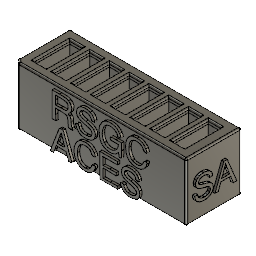
Bargraph Updated 8 Pin (Autodesk Fusion 360 design; units mm, degrees)
Autodesk Fusion 360 part; units mm, degrees
note: some values were not read from the file. Chosen so that the rebuilt part matches the saved one: which face or edge a step refers to; which pieces of a blend or face edit are solid. Set by a fixed rule: which sketch regions a step uses.
(part 1 of 2)
sketch "Sketch2" plane through (0, 0, 0) normal (0, 0, 1) x (-1, 0, 0)
  line L0 (0, -5.1) -> (-2.1, -5.1)
  line L1 (-2.1, -5.1) -> (-2.1, 0)
  line L2 (-2.1, 0) -> (0, 0)
  line L3 (0, 0) -> (0, -5.1)
  line L4 (-2.54, -5.1) -> (-2.54, 0)
  line L5 (-4.64, -5.1) -> (-2.54, -5.1)
  line L6 (-4.64, 0) -> (-4.64, -5.1)
  line L7 (-2.54, 0) -> (-4.64, 0)
  line L8 (-1.05, -2.55) -> (-1.05, -1.28)
  line L9 (-1.05, -2.55) -> (-1.05, -3.82)
  line L10 (-1.05, -3.82) -> (-3.59, -3.82)
  line L11 (-7.62, 0) -> (-9.72, 0)
  line L12 (-5.08, -5.1) -> (-7.18, -5.1)
  line L13 (-7.18, 0) -> (-5.08, 0)
  line L14 (-7.18, -5.1) -> (-7.18, 0)
  line L15 (-7.62, -5.1) -> (-7.62, 0)
  line L16 (-9.72, 0) -> (-9.72, -5.1)
  line L17 (-9.72, -5.1) -> (-7.62, -5.1)
  line L18 (-5.08, 0) -> (-5.08, -5.1)
  line L19 (-7.18, -2.55) -> (-6.13, -2.55)
  line L20 (-6.13, -2.55) -> (-6.13, -3.82)
  line L21 (-3.59, -3.82) -> (-6.13, -3.82)
  line L22 (-9.72, -2.55) -> (-8.67, -2.55)
  line L23 (-8.67, -2.55) -> (-8.67, -3.82)
  line L24 (-8.67, -3.82) -> (-11.21, -3.82)
  line L25 (-12.26, -5.1) -> (-12.26, 0)
  line L26 (-16.29, -2.55) -> (-16.29, -3.82)
  line L27 (-11.21, -3.82) -> (-13.75, -3.82)
  line L28 (-17.78, 0) -> (-19.88, 0)
  line L29 (-17.34, -2.55) -> (-16.29, -2.55)
  line L30 (-19.88, 0) -> (-19.88, -5.1)
  line L31 (-14.8, 0) -> (-14.8, -5.1)
  line L32 (-17.34, -5.1) -> (-17.34, 0)
  line L33 (-12.7, 0) -> (-14.8, 0)
  line L34 (-11.21, -2.55) -> (-11.21, -3.82)
  line L35 (-10.16, -5.1) -> (-12.26, -5.1)
  line L36 (-15.24, -5.1) -> (-17.34, -5.1)
  line L37 (-15.24, 0) -> (-15.24, -5.1)
  line L38 (-14.8, -5.1) -> (-12.7, -5.1)
  line L39 (-12.7, -5.1) -> (-12.7, 0)
  line L40 (-17.34, 0) -> (-15.24, 0)
  line L41 (-10.16, 0) -> (-10.16, -5.1)
  line L42 (-11.21, -2.55) -> (-11.21, -1.28)
  line L43 (-13.75, -3.82) -> (-16.29, -3.82)
  line L44 (-17.78, -5.1) -> (-17.78, 0)
  line L45 (-12.26, 0) -> (-10.16, 0)
  line L46 (-19.88, -5.1) -> (-17.78, -5.1)
  line L47 (-18.83, -2.55) -> (-18.83, -3.82)
  line L48 (-19.88, -2.55) -> (-18.83, -2.55)
  line L49 (0, 0) -> (0, 1)
  line L50 (0, 1) -> (1, 1)
  line L51 (-20.04, -5.1) -> (-21.04, -5.1)
  line L52 (-21.04, -5.1) -> (-21.04, -6.1)
  line L53 (-21.04, -6.1) -> (1, -6.1)
  line L54 (1, -6.1) -> (1, 1)
  line L55 (1, 1) -> (-21.04, 1)
  line L56 (-21.04, 1) -> (-21.04, -6.1)
  line L57 (0.5, 0.5) -> (-20.54, 0.5)
  line L58 (-20.54, 0.5) -> (-20.54, -5.6)
  line L59 (-20.54, -5.6) -> (0.5, -5.6)
  line L60 (0.5, -5.6) -> (0.5, 0.5)
  point P0 (-21.37, -3.82)
  point P1 (-26.45, -3.82)
  point P2 (-26.45, -3.82)
  dimension "d8" = 2.1
  dimension "d9" = 5.1
  dimension "d18" = 1.27
  dimension "d19" = 1.27
  dimension "d29" = 1.05
  dimension "d30" = 2.54
  dimension "d31" = 1.05
  dimension "d32" = 2.54
  dimension "d33" = 2.1
  dimension "d34" = 5.1
  dimension "d35" = 1.27
  dimension "d36" = 1.27
  dimension "d37" = 1.05
  dimension "d38" = 2.54
  dimension "d39" = 1.05
  dimension "d46" = 1
  dimension "d47" = 1
  dimension "d48" = 1
  dimension "d49" = 1
  dimension "d92" = -0.5
  dimension "d95" = 21.04
  dimension "d96" = 6.1
  constraint horizontal L0
  constraint vertical L1
  constraint horizontal L2
  constraint vertical L3
  constraint perpendicular L2 L8
  constraint parallel L8 L9
  constraint perpendicular L4 L10
  constraint horizontal L12
  constraint vertical L14
  constraint horizontal L13
  constraint vertical L18
  constraint midpoint L14 L19.start
  constraint perpendicular L18 L19
  constraint perpendicular L10 L20
  constraint perpendicular L18 L21
  constraint midpoint L16 L22.start
  constraint perpendicular L16 L22
  constraint perpendicular L21 L23
  constraint perpendicular L23 L24
  constraint horizontal L35
  constraint vertical L25
  constraint horizontal L45
  constraint vertical L41
  constraint perpendicular L42 L45
  constraint parallel L34 L42
  constraint perpendicular L27 L39
  constraint horizontal L36
  constraint vertical L32
  constraint horizontal L40
  constraint vertical L37
  constraint midpoint L29.start L32
  constraint perpendicular L29 L37
  constraint perpendicular L26 L27
  constraint perpendicular L37 L43
  constraint midpoint L48.start L30
  constraint perpendicular L30 L48
  constraint perpendicular L43 L47
  constraint perpendicular L2 L49
  constraint perpendicular L3 L50
  constraint horizontal L53
  constraint vertical L54
  constraint horizontal L55
  constraint vertical L56
  measures "d8" distance of L0.start L0.end
  measures "d9" distance of L0.start L2.end
  measures "d18" distance of L8.start L8.end
  measures "d19" distance of L8.start L9.end
  measures "d29" distance of L19.start L19.end
  measures "d30" distance of L10.end L20.end
  measures "d31" distance of L22.start L22.end
  measures "d32" distance of L23.end L24.end
  measures "d33" distance of L35.start L25.start
  measures "d34" distance of L35.start L41.start
  measures "d35" distance of L42.end L34.start
  measures "d36" distance of L24.end L34.start
  measures "d37" distance of L26.start L29.start
  measures "d38" distance of L27.end L26.end
  measures "d39" distance of L48.start L47.start
  measures "d46" distance of L2.end L49.end
  measures "d47" distance of L49.end L50.end
  measures "d48" distance of L51.start L51.end
  measures "d49" distance of L51.end L52.end
  measures "d95" distance of L57.start L57.end
  measures "d96" distance of L57.start L59.end
extrude "Extrude5" add sketch "Sketch2" along normal blind 7.5
sketch "Sketch5" plane through (0, 0, 7.5) normal (0, 0, 1) x (-1, 0, 0)
  line L0 (-17.78, -5.1) -> (-19.88, -5.1)
  line L1 (-19.88, -5.1) -> (-19.88, 0)
  line L2 (-19.88, 0) -> (-17.78, 0)
  line L3 (-17.78, 0) -> (-17.78, -5.1)
  line L4 (-7.18, 0) -> (-5.08, 0)
  line L5 (-5.08, 0) -> (-5.08, -5.1)
  line L6 (-5.08, -5.1) -> (-7.18, -5.1)
  line L7 (-7.18, -5.1) -> (-7.18, 0)
  line L8 (-2.1, 0) -> (0, 0)
  line L9 (0, 0) -> (0, -5.1)
  line L10 (0, -5.1) -> (-2.1, -5.1)
  line L11 (-2.1, -5.1) -> (-2.1, 0)
  line L12 (-17.34, -5.1) -> (-17.34, 0)
  line L13 (-17.34, 0) -> (-15.24, 0)
  line L14 (-15.24, 0) -> (-15.24, -5.1)
  line L15 (-15.24, -5.1) -> (-17.34, -5.1)
  line L16 (-12.7, 0) -> (-12.7, -5.1)
  line L17 (-12.7, -5.1) -> (-14.8, -5.1)
  line L18 (-14.8, -5.1) -> (-14.8, 0)
  line L19 (-14.8, 0) -> (-12.7, 0)
  line L20 (-12.26, -5.1) -> (-12.26, 0)
  line L21 (-12.26, 0) -> (-10.16, 0)
  line L22 (-10.16, 0) -> (-10.16, -5.1)
  line L23 (-10.16, -5.1) -> (-12.26, -5.1)
  line L24 (-7.62, -5.1) -> (-9.72, -5.1)
  line L25 (-9.72, -5.1) -> (-9.72, 0)
  line L26 (-9.72, 0) -> (-7.62, 0)
  line L27 (-7.62, 0) -> (-7.62, -5.1)
  line L28 (-4.64, 0) -> (-2.54, 0)
  line L29 (-2.54, 0) -> (-2.54, -5.1)
  line L30 (-2.54, -5.1) -> (-4.64, -5.1)
  line L31 (-4.64, -5.1) -> (-4.64, 0)
  line L32 (-21.04, 1) -> (-21.04, -6.1)
  line L33 (-21.04, -6.1) -> (1, -6.1)
  line L34 (1, -6.1) -> (1, 1)
  line L35 (1, 1) -> (-21.04, 1)
  line L36 (-18.83, -2.55) -> (-16.29, -2.55)
  line L37 (-16.29, -2.55) -> (-13.75, -2.55)
  line L38 (-13.75, -2.55) -> (-11.21, -2.55)
  line L39 (-11.21, -2.55) -> (-8.67, -2.55)
  line L40 (-8.67, -2.55) -> (-6.13, -2.55)
  line L41 (-6.13, -2.55) -> (-3.59, -2.55)
  line L42 (-3.59, -2.55) -> (-1.05, -2.55)
  line L43 (-0.25, -4.85) -> (-1.85, -4.85)
  line L44 (-1.85, -4.85) -> (-1.85, -0.25)
  line L45 (-1.85, -0.25) -> (-0.25, -0.25)
  line L46 (-0.25, -0.25) -> (-0.25, -4.85)
  line L47 (-0.25, -4.85) -> (-1.85, -0.25) construction
  line L48 (-1.85, -4.85) -> (-0.25, -0.25) construction
  line L49 (-2.79, -4.85) -> (-4.39, -4.85)
  line L50 (-2.79, -0.25) -> (-2.79, -4.85)
  line L51 (-4.39, -0.25) -> (-2.79, -0.25)
  line L52 (-4.39, -4.85) -> (-4.39, -0.25)
  line L53 (-5.33, -0.25) -> (-5.33, -4.85)
  line L54 (-5.33, -4.85) -> (-6.93, -4.85)
  line L55 (-6.93, -0.25) -> (-5.33, -0.25)
  line L56 (-6.93, -4.85) -> (-6.93, -0.25)
  line L57 (-9.47, -0.25) -> (-7.87, -0.25)
  line L58 (-7.87, -0.25) -> (-7.87, -4.85)
  line L59 (-7.87, -4.85) -> (-9.47, -4.85)
  line L60 (-9.47, -4.85) -> (-9.47, -0.25)
  line L61 (-10.41, -0.25) -> (-10.41, -4.85)
  line L62 (-12.01, -0.25) -> (-10.41, -0.25)
  line L63 (-12.01, -4.85) -> (-12.01, -0.25)
  line L64 (-10.41, -4.85) -> (-12.01, -4.85)
  line L65 (-12.95, -4.85) -> (-14.55, -4.85)
  line L66 (-14.55, -0.25) -> (-12.95, -0.25)
  line L67 (-14.55, -4.85) -> (-14.55, -0.25)
  line L68 (-12.95, -0.25) -> (-12.95, -4.85)
  line L69 (-15.49, -4.85) -> (-17.09, -4.85)
  line L70 (-15.49, -0.25) -> (-15.49, -4.85)
  line L71 (-17.09, -0.25) -> (-15.49, -0.25)
  line L72 (-17.09, -4.85) -> (-17.09, -0.25)
  line L73 (-19.63, -4.85) -> (-19.63, -0.25)
  line L74 (-18.03, -4.85) -> (-19.63, -4.85)
  line L75 (-19.63, -0.25) -> (-18.03, -0.25)
  line L76 (-18.03, -0.25) -> (-18.03, -4.85)
  line L77 (1, 1) -> (-31.04, 1)
  line L78 (-31.04, 1) -> (-31.04, -6.1)
  line L79 (-31.04, -6.1) -> (1, -6.1)
  line L80 (1, -6.1) -> (1, 1)
  line L81 (-30.54, 1) -> (-31.04, 0.4867)
  point P0 (-1.05, -2.55)
  point P1 (-6.13, -2.55)
  point P2 (-8.67, -2.55)
  point P3 (-8.67, -2.55)
  point P4 (-11.21, -2.55)
  point P5 (-11.21, -2.55)
  point P6 (-11.21, -2.55)
  point P7 (-13.75, -2.55)
  point P8 (-13.75, -2.55)
  point P9 (-13.75, -2.55)
  point P10 (-13.75, -2.55)
  point P11 (-16.29, -2.55)
  point P12 (-16.29, -2.55)
  point P13 (-16.29, -2.55)
  point P14 (-16.29, -2.55)
  point P15 (-16.29, -2.55)
  point P16 (-18.83, -2.55)
  point P17 (-18.83, -2.55)
  point P18 (-18.83, -2.55)
  point P19 (-18.83, -2.55)
  point P20 (-18.83, -2.55)
  point P21 (-18.83, -2.55)
  point P22 (-21.37, -2.55)
  point P23 (-21.37, -2.55)
  point P24 (-21.37, -2.55)
  point P25 (-21.37, -2.55)
  point P26 (-21.37, -2.55)
  point P27 (-21.37, -2.55)
  point P28 (-23.91, -2.55)
  point P29 (-23.91, -2.55)
  point P30 (-23.91, -2.55)
  point P31 (-23.91, -2.55)
  point P32 (-23.91, -2.55)
  point P33 (-23.91, -2.55)
  point P34 (-23.91, -2.55)
  point P35 (-23.91, -2.55)
  point P36 (-26.45, -2.55)
  point P37 (-26.45, -2.55)
  point P38 (-26.45, -2.55)
  point P39 (-26.45, -2.55)
  point P40 (-26.45, -2.55)
  point P41 (-26.45, -2.55)
  point P42 (-26.45, -2.55)
  point P43 (-26.45, -2.55)
  point P44 (-26.45, -2.55)
  point P45 (-28.99, -2.55)
  point P46 (-28.99, -2.55)
  point P47 (-28.99, -2.55)
  point P48 (-28.99, -2.55)
  point P49 (-28.99, -2.55)
  point P50 (-28.99, -2.55)
  point P51 (-28.99, -2.55)
  point P52 (-28.99, -2.55)
  point P53 (-28.99, -2.55)
  point P54 (-28.99, -2.55)
  dimension "d57" = 2.54
  dimension "d58" = 2.54
  dimension "d59" = 2.54
  dimension "d60" = 2.54
  dimension "d61" = 2.54
  dimension "d62" = 2.54
  dimension "d63" = 2.54
  dimension "d64" = 1.6
  dimension "d65" = 4.6
  dimension "d66" = 1.6
  dimension "d67" = 4.6
  dimension "d68" = 1.6
  dimension "d69" = 4.6
  dimension "d70" = 1.6
  dimension "d71" = 4.6
  dimension "d72" = 1.6
  dimension "d73" = 4.6
  dimension "d74" = 1.6
  dimension "d75" = 4.6
  dimension "d76" = 1.6
  dimension "d77" = 4.6
  dimension "d78" = 1.6
  dimension "d79" = 4.6
  constraint perpendicular L1 L36
  constraint perpendicular L18 L37
  constraint perpendicular L20 L38
  constraint perpendicular L25 L39
  constraint perpendicular L7 L40
  constraint perpendicular L31 L41
  constraint perpendicular L11 L42
  constraint horizontal L43
  constraint perpendicular L43 L44
  constraint parallel L43 L45
  constraint parallel L44 L46
  constraint coincident L47 P0
  constraint coincident L48 P0
  constraint coincident P0 L42.end
  constraint horizontal L49
  constraint perpendicular L49 L52
  constraint parallel L49 L51
  constraint parallel L50 L52
  constraint horizontal L54
  constraint perpendicular L54 L56
  constraint parallel L54 L55
  constraint parallel L53 L56
  constraint horizontal L59
  constraint perpendicular L59 L60
  constraint parallel L57 L59
  constraint parallel L58 L60
  constraint horizontal L64
  constraint perpendicular L63 L64
  constraint parallel L62 L64
  constraint parallel L61 L63
  constraint horizontal L65
  constraint perpendicular L65 L67
  constraint parallel L65 L66
  constraint parallel L67 L68
  constraint horizontal L69
  constraint perpendicular L69 L72
  constraint parallel L69 L71
  constraint parallel L70 L72
  constraint horizontal L74
  constraint perpendicular L73 L74
  constraint parallel L74 L75
  constraint parallel L73 L76
  constraint horizontal L77
  constraint vertical L78
  constraint horizontal L79
  constraint vertical L80
  constraint coincident L32.end L78.end
  constraint coincident L34.end L35.start
  constraint coincident L32.start L81.start
  constraint coincident L32.start L81.end
  measures "d57" distance of P21 P15
  measures "d58" distance of P15 P10
  measures "d59" distance of P10 P6
  measures "d60" distance of P6 P3
  measures "d61" distance of P3 P1
  measures "d62" distance of P1 L41.end
  measures "d63" distance of L41.end P0
  measures "d64" distance of L44.end L45.end
  measures "d65" distance of L43.end L44.end
  measures "d66" distance of L51.start L50.start
  measures "d67" distance of L49.end L51.start
  measures "d68" distance of L53.start L55.start
  measures "d69" distance of L54.end L55.start
  measures "d70" distance of L57.start L57.end
  measures "d71" distance of L57.start L59.end
  measures "d72" distance of L62.start L61.start
  measures "d73" distance of L62.start L63.start
  measures "d74" distance of L66.start L66.end
  measures "d75" distance of L66.start L65.end
  measures "d76" distance of L71.start L70.start
  measures "d77" distance of L71.start L69.end
  measures "d78" distance of L73.end L75.end
  measures "d79" distance of L73.start L73.end
extrude "Extrude6" add sketch "Sketch5" along normal blind 0.7 contours L0 L1 L2 L3 | L4 L5 L7 L40 L41 L53 L55 L56 | L5 L6 L7 L40 L41 L53 L54 L56 | L8 L9 L10 L11 | L12 L14 L15 L36 L37 L69 L70 L72 | L12 L13 L14 L36 L37 L70 L71 L72 | L16 L18 L19 L37 L38 L66 L67 L68 | L16 L17 L18 L37 L38 L65 L67 L68 | L20 L22 L23 L38 L39 L61 L63 L64 | L20 L21 L22 L38 L39 L61 L62 L63 | L24 L25 L27 L39 L40 L58 L59 L60 | L25 L26 L27 L39 L40 L57 L58 L60 | L28 L29 L31 L41 L42 L50 L51 L52 | L29 L30 L31 L41 L42 L49 L50 L52
extrude "Extrude7" add sketch "Sketch5" along normal blind 0.2 contours L32 L33 L34 L35 L77 L79 L80
sketch "Sketch7" plane through (0, 0, 0) normal (0, 0, 1) x (1, 0, 0)
  line L0 (0, 0) -> (-0.5, 0)
  line L1 (-0.5, 0) -> (-0.5, -0.5)
  line L2 (-0.5, -0.5) -> (20.74, -0.5)
  line L3 (20.74, -0.5) -> (20.74, 5.6)
  line L4 (20.74, 5.6) -> (-0.5, 5.6)
  line L5 (-0.5, 5.6) -> (-0.5, -0.5)
  dimension "d93" = 0.5
  dimension "d94" = 0.5
  dimension "d97" = 21.24
  dimension "d98" = 6.1
  constraint coincident L0.start origin
  constraint horizontal L0
  constraint perpendicular L0 L1
  constraint horizontal L2
  constraint vertical L3
  constraint horizontal L4
  constraint vertical L5
  measures "d93" distance of L0.start L0.end
  measures "d94" distance of L0.end L1.end
  measures "d97" distance of L1.end L2.end
  measures "d98" distance of L1.end L4.end
extrude "Extrude8" cut sketch "Sketch7" along normal blind 0.5
sketch "Sketch8" plane through (0, -1, 0) normal (0, -1, 0) x (1, 0, 0)
  line L0 (-1, 0) -> (21.04, 0)
  line L1 (21.04, 7.7) -> (-1, 7.7)
  line L2 (-1, 7.7) -> (-1, 0)
  line L3 (21.04, 0) -> (21.04, 7.7)
  line L4 (10.02, 7.7) -> (10.02, 0) construction
  line L5 (-1, 3.85) -> (21.04, 3.85) construction
  spline S0 degree 3 poles (7.6982, 7.3236) (7.3931, 7.1177) (7.2482, 6.866) (7.2482, 6.5227) knots 0 0 0 0 1 1 1 1
  spline S1 degree 3 poles (7.2482, 6.5227) (7.2482, 6.1261) (7.5533, 5.8744) (8.2398, 5.7066) knots 0 0 0 0 1 1 1 1
  spline S2 degree 3 poles (8.2398, 5.7066) (9.0864, 5.5083) (9.2313, 5.4168) (9.2313, 5.0964) knots 0 0 0 0 1 1 1 1
  spline S3 degree 3 poles (9.2313, 5.0964) (9.2313, 4.7684) (8.9949, 4.593) (8.4838, 4.5473) knots 0 0 0 0 1 1 1 1
  spline S4 degree 3 poles (8.4838, 4.5473) (8.0262, 4.5091) (7.6677, 4.7151) (7.5915, 5.0583) knots 0 0 0 0 1 1 1 1
  spline S5 degree 3 poles (7.5915, 5.0583) (7.5457, 5.2566) (7.5076, 5.2947) (7.3398, 5.2718) knots 0 0 0 0 1 1 1 1
  spline S6 degree 3 poles (7.3398, 5.2718) (7.172, 5.2566) (7.1414, 5.2185) (7.1567, 5.0583) knots 0 0 0 0 1 1 1 1
  spline S7 degree 3 poles (7.1567, 5.0583) (7.1872, 4.8218) (7.3779, 4.5473) (7.6601, 4.3413) knots 0 0 0 0 1 1 1 1
  spline S8 degree 3 poles (7.6601, 4.3413) (7.8279, 4.2117) (7.9728, 4.1811) (8.3847, 4.1888) knots 0 0 0 0 1 1 1 1
  spline S9 degree 3 poles (8.3847, 4.1888) (9.1398, 4.204) (9.5745, 4.4786) (9.6584, 4.9896) knots 0 0 0 0 1 1 1 1
  spline S10 degree 3 poles (9.6584, 4.9896) (9.7576, 5.5846) (9.4449, 5.8668) (8.461, 6.088) knots 0 0 0 0 1 1 1 1
  spline S11 degree 3 poles (8.461, 6.088) (7.7593, 6.2481) (7.5686, 6.4159) (7.6982, 6.7592) knots 0 0 0 0 1 1 1 1
  spline S12 degree 3 poles (7.6982, 6.7592) (7.7974, 7.0185) (8.0033, 7.1177) (8.4305, 7.1177) knots 0 0 0 0 1 1 1 1
  spline S13 degree 3 poles (8.4305, 7.1177) (8.6974, 7.1177) (8.8194, 7.0719) (8.9644, 6.927) knots 0 0 0 0 1 1 1 1
  spline S14 degree 3 poles (8.9644, 6.927) (9.0711, 6.8278) (9.155, 6.6905) (9.155, 6.6219) knots 0 0 0 0 1 1 1 1
  spline S15 degree 3 poles (9.155, 6.6219) (9.155, 6.5456) (9.2313, 6.5075) (9.3839, 6.5075) knots 0 0 0 0 1 1 1 1
  spline S16 degree 3 poles (9.3839, 6.5075) (9.5974, 6.5075) (9.6127, 6.5227) (9.5669, 6.721) knots 0 0 0 0 1 1 1 1
  spline S17 degree 3 poles (9.5669, 6.721) (9.483, 7.0566) (9.3152, 7.2473) (8.9949, 7.377) knots 0 0 0 0 1 1 1 1
  spline S18 degree 3 poles (8.9949, 7.377) (8.5525, 7.56) (8.011, 7.5372) (7.6982, 7.3236) knots 0 0 0 0 1 1 1 1
  spline S19 degree 3 poles (10.9017, 7.3236) (10.65, 7.1863) (10.5127, 7.0414) (10.3525, 6.7287) knots 0 0 0 0 1 1 1 1
  spline S20 degree 3 poles (10.3525, 6.7287) (10.1542, 6.3549) (10.1313, 6.2634) (10.1618, 5.699) knots 0 0 0 0 1 1 1 1
  spline S21 degree 3 poles (10.1618, 5.699) (10.2, 4.9973) (10.3678, 4.6312) (10.7797, 4.3871) knots 0 0 0 0 1 1 1 1
  spline S22 degree 3 poles (10.7797, 4.3871) (11.2907, 4.082) (12.061, 4.1278) (12.4424, 4.4939) knots 0 0 0 0 1 1 1 1
  line L6 (12.4424, 4.4939) -> (12.6407, 4.6845)
  line L7 (12.6407, 4.6845) -> (12.6865, 4.4557)
  spline S23 degree 3 poles (12.6865, 4.4557) (12.7246, 4.2879) (12.778, 4.2193) (12.8924, 4.2193) knots 0 0 0 0 1 1 1 1
  spline S24 degree 3 poles (12.8924, 4.2193) (13.0373, 4.2193) (13.045, 4.265) (13.045, 5.0964) knots 0 0 0 0 1 1 1 1
  line L8 (13.045, 5.0964) -> (13.045, 5.9736)
  line L9 (13.045, 5.9736) -> (12.3204, 5.9736)
  spline S25 degree 3 poles (12.3204, 5.9736) (11.5958, 5.9736) (11.5958, 5.9736) (11.5958, 5.7829) knots 0 0 0 0 1 1 1 1
  spline S26 degree 3 poles (11.5958, 5.7829) (11.5958, 5.5998) (11.611, 5.5922) (12.1221, 5.5922) knots 0 0 0 0 1 1 1 1
  line L10 (12.1221, 5.5922) -> (12.6483, 5.5922)
  line L11 (12.6483, 5.5922) -> (12.5797, 5.31)
  spline S27 degree 3 poles (12.5797, 5.31) (12.4043, 4.5244) (11.2907, 4.2727) (10.8178, 4.9134) knots 0 0 0 0 1 1 1 1
  spline S28 degree 3 poles (10.8178, 4.9134) (10.3678, 5.5159) (10.5508, 6.7134) (11.1458, 7.0185) knots 0 0 0 0 1 1 1 1
  spline S29 degree 3 poles (11.1458, 7.0185) (11.6034, 7.2549) (12.3814, 7.0261) (12.4805, 6.6219) knots 0 0 0 0 1 1 1 1
  spline S30 degree 3 poles (12.4805, 6.6219) (12.5187, 6.477) (12.5721, 6.4312) (12.7475, 6.4312) knots 0 0 0 0 1 1 1 1
  spline S31 degree 3 poles (12.7475, 6.4312) (13.0145, 6.4312) (13.0221, 6.5075) (12.8009, 6.8965) knots 0 0 0 0 1 1 1 1
  spline S32 degree 3 poles (12.8009, 6.8965) (12.4729, 7.4761) (11.5805, 7.6821) (10.9017, 7.3236) knots 0 0 0 0 1 1 1 1
  spline S33 degree 3 poles (14.4179, 7.4151) (13.8763, 7.2016) (13.556, 6.6143) (13.556, 5.8591) knots 0 0 0 0 1 1 1 1
  spline S34 degree 3 poles (13.556, 5.8591) (13.5636, 4.7608) (14.0365, 4.1964) (14.9518, 4.1964) knots 0 0 0 0 1 1 1 1
  spline S35 degree 3 poles (14.9518, 4.1964) (15.1959, 4.1964) (15.4781, 4.2498) (15.6154, 4.3184) knots 0 0 0 0 1 1 1 1
  spline S36 degree 3 poles (15.6154, 4.3184) (15.9205, 4.4786) (16.2332, 4.8829) (16.2942, 5.1956) knots 0 0 0 0 1 1 1 1
  spline S37 degree 3 poles (16.2942, 5.1956) (16.34, 5.4168) (16.3247, 5.4396) (16.1493, 5.4396) knots 0 0 0 0 1 1 1 1
  spline S38 degree 3 poles (16.1493, 5.4396) (15.9891, 5.4396) (15.9205, 5.3786) (15.7984, 5.104) knots 0 0 0 0 1 1 1 1
  spline S39 degree 3 poles (15.7984, 5.104) (15.7221, 4.921) (15.5696, 4.7227) (15.4704, 4.6693) knots 0 0 0 0 1 1 1 1
  spline S40 degree 3 poles (15.4704, 4.6693) (15.2187, 4.532) (14.6925, 4.5549) (14.456, 4.7074) knots 0 0 0 0 1 1 1 1
  spline S41 degree 3 poles (14.456, 4.7074) (14.1357, 4.921) (13.9374, 5.4549) (13.9831, 5.9736) knots 0 0 0 0 1 1 1 1
  spline S42 degree 3 poles (13.9831, 5.9736) (14.0518, 6.7668) (14.3797, 7.1177) (15.0433, 7.1177) knots 0 0 0 0 1 1 1 1
  spline S43 degree 3 poles (15.0433, 7.1177) (15.4247, 7.1177) (15.6688, 6.9727) (15.8289, 6.6524) knots 0 0 0 0 1 1 1 1
  spline S44 degree 3 poles (15.8289, 6.6524) (15.9128, 6.4998) (16.0044, 6.4312) (16.134, 6.4312) knots 0 0 0 0 1 1 1 1
  spline S45 degree 3 poles (16.134, 6.4312) (16.3705, 6.4312) (16.3705, 6.5151) (16.1645, 6.8888) knots 0 0 0 0 1 1 1 1
  spline S46 degree 3 poles (16.1645, 6.8888) (15.9433, 7.2855) (15.5315, 7.499) (15.0204, 7.4914) knots 0 0 0 0 1 1 1 1
  spline S47 degree 3 poles (15.0204, 7.4914) (14.7916, 7.4914) (14.5247, 7.4533) (14.4179, 7.4151) knots 0 0 0 0 1 1 1 1
  line L12 (4.121, 5.821) -> (4.121, 4.2193)
  line L13 (4.121, 4.2193) -> (4.3575, 4.2193)
  line L14 (4.3575, 4.2193) -> (4.5939, 4.2193)
  line L15 (4.5939, 4.2193) -> (4.571, 4.921)
  line L16 (4.571, 4.921) -> (4.5405, 5.6227)
  line L17 (4.5405, 5.6227) -> (5.227, 5.5998)
  spline S48 degree 3 poles (5.227, 5.5998) (5.6618, 5.5922) (5.9516, 5.5464) (6.0126, 5.4778) knots 0 0 0 0 1 1 1 1
  spline S49 degree 3 poles (6.0126, 5.4778) (6.0736, 5.4244) (6.1423, 5.1269) (6.1652, 4.8218) knots 0 0 0 0 1 1 1 1
  line L18 (6.1652, 4.8218) -> (6.2185, 4.2574)
  line L19 (6.2185, 4.2574) -> (6.5084, 4.2345)
  spline S50 degree 3 poles (6.5084, 4.2345) (6.8135, 4.2117) (6.844, 4.2574) (6.6762, 4.4786) knots 0 0 0 0 1 1 1 1
  spline S51 degree 3 poles (6.6762, 4.4786) (6.6075, 4.5701) (6.5618, 4.799) (6.5618, 5.0659) knots 0 0 0 0 1 1 1 1
  spline S52 degree 3 poles (6.5618, 5.0659) (6.5618, 5.4473) (6.5313, 5.5235) (6.3711, 5.6532) knots 0 0 0 0 1 1 1 1
  line L20 (6.3711, 5.6532) -> (6.1804, 5.8058)
  line L21 (6.1804, 5.8058) -> (6.4092, 6.0346)
  spline S53 degree 3 poles (6.4092, 6.0346) (6.7753, 6.4083) (6.6991, 6.988) (6.2414, 7.2702) knots 0 0 0 0 1 1 1 1
  spline S54 degree 3 poles (6.2414, 7.2702) (6.0279, 7.3999) (5.8524, 7.4227) (5.0592, 7.4227) knots 0 0 0 0 1 1 1 1
  line L22 (5.0592, 7.4227) -> (4.121, 7.4227)
  line L23 (4.121, 7.4227) -> (4.121, 5.821)
  spline S55 degree 3 poles (6.0507, 6.9117) (6.2109, 6.7668) (6.2185, 6.3625) (6.0736, 6.1566) knots 0 0 0 0 1 1 1 1
  spline S56 degree 3 poles (6.0736, 6.1566) (5.9821, 6.0346) (5.8524, 6.0041) (5.2499, 5.9888) knots 0 0 0 0 1 1 1 1
  line L24 (5.2499, 5.9888) -> (4.5405, 5.9583)
  line L25 (4.5405, 5.9583) -> (4.5482, 6.5227)
  spline S57 degree 2 poles (4.5482, 6.5227) (4.5558, 6.8278) (4.571, 7.0795) knots 0 0 0 1 1 1
  spline S58 degree 3 poles (4.571, 7.0795) (5.3261, 7.0795) (5.9363, 7.0109) (6.0507, 6.9117) knots 0 0 0 0 1 1 1 1
  spline S59 degree 3 poles (7.78, 3.6111) (6.93, 3.2383) (6.6467, 1.9037) (7.2431, 1.0239) knots 0 0 0 0 1 1 1 1
  spline S60 degree 3 poles (7.2431, 1.0239) (7.4892, 0.6511) (7.8322, 0.487) (8.3466, 0.487) knots 0 0 0 0 1 1 1 1
  spline S61 degree 3 poles (8.3466, 0.487) (8.876, 0.487) (9.301, 0.7331) (9.5321, 1.1804) knots 0 0 0 0 1 1 1 1
  spline S62 degree 3 poles (9.5321, 1.1804) (9.7409, 1.5905) (9.726, 1.7024) (9.4576, 1.7024) knots 0 0 0 0 1 1 1 1
  spline S63 degree 3 poles (9.4576, 1.7024) (9.2861, 1.7024) (9.2339, 1.6725) (9.2339, 1.5532) knots 0 0 0 0 1 1 1 1
  spline S64 degree 3 poles (9.2339, 1.5532) (9.2339, 1.4712) (9.1221, 1.2774) (8.9879, 1.1282) knots 0 0 0 0 1 1 1 1
  spline S65 degree 3 poles (8.9879, 1.1282) (8.7642, 0.8896) (8.6896, 0.8598) (8.3839, 0.8598) knots 0 0 0 0 1 1 1 1
  spline S66 degree 3 poles (8.3839, 0.8598) (7.7576, 0.8598) (7.3699, 1.3221) (7.3699, 2.0752) knots 0 0 0 0 1 1 1 1
  spline S67 degree 3 poles (7.3699, 2.0752) (7.3774, 2.8879) (7.7502, 3.3427) (8.4287, 3.3427) knots 0 0 0 0 1 1 1 1
  spline S68 degree 3 poles (8.4287, 3.3427) (8.8089, 3.3427) (9.0326, 3.2085) (9.1593, 2.8953) knots 0 0 0 0 1 1 1 1
  spline S69 degree 3 poles (9.1593, 2.8953) (9.2339, 2.7164) (9.301, 2.6716) (9.465, 2.6716) knots 0 0 0 0 1 1 1 1
  spline S70 degree 3 poles (9.465, 2.6716) (9.726, 2.6716) (9.7409, 2.7835) (9.5098, 3.1265) knots 0 0 0 0 1 1 1 1
  spline S71 degree 3 poles (9.5098, 3.1265) (9.2339, 3.5365) (8.9058, 3.7155) (8.4212, 3.7155) knots 0 0 0 0 1 1 1 1
  spline S72 degree 3 poles (8.4212, 3.7155) (8.1901, 3.708) (7.8993, 3.6633) (7.78, 3.6111) knots 0 0 0 0 1 1 1 1
  spline S73 degree 3 poles (13.5882, 3.6409) (13.29, 3.5216) (13.0365, 3.1339) (13.0365, 2.7909) knots 0 0 0 0 1 1 1 1
  spline S74 degree 3 poles (13.0365, 2.7909) (13.0365, 2.3436) (13.2527, 2.1721) (14.0505, 1.9559) knots 0 0 0 0 1 1 1 1
  spline S75 degree 3 poles (14.0505, 1.9559) (14.7514, 1.7695) (14.975, 1.6203) (14.975, 1.3519) knots 0 0 0 0 1 1 1 1
  spline S76 degree 3 poles (14.975, 1.3519) (14.975, 0.9866) (14.4531, 0.7331) (13.8939, 0.8375) knots 0 0 0 0 1 1 1 1
  spline S77 degree 3 poles (13.8939, 0.8375) (13.618, 0.8896) (13.3347, 1.1804) (13.3347, 1.4116) knots 0 0 0 0 1 1 1 1
  spline S78 degree 3 poles (13.3347, 1.4116) (13.3347, 1.516) (13.2825, 1.5532) (13.111, 1.5532) knots 0 0 0 0 1 1 1 1
  spline S79 degree 3 poles (13.111, 1.5532) (12.8501, 1.5532) (12.8426, 1.516) (13.0066, 1.1059) knots 0 0 0 0 1 1 1 1
  spline S80 degree 3 poles (13.0066, 1.1059) (13.1334, 0.7853) (13.4316, 0.5616) (13.8343, 0.4721) knots 0 0 0 0 1 1 1 1
  spline S81 degree 3 poles (13.8343, 0.4721) (14.1549, 0.405) (14.8408, 0.5541) (15.0794, 0.7405) knots 0 0 0 0 1 1 1 1
  spline S82 degree 3 poles (15.0794, 0.7405) (15.3478, 0.9568) (15.4597, 1.3967) (15.318, 1.7322) knots 0 0 0 0 1 1 1 1
  spline S83 degree 3 poles (15.318, 1.7322) (15.1913, 2.0453) (14.9676, 2.1646) (14.2369, 2.3287) knots 0 0 0 0 1 1 1 1
  spline S84 degree 3 poles (14.2369, 2.3287) (13.6255, 2.4629) (13.4093, 2.6045) (13.4093, 2.8655) knots 0 0 0 0 1 1 1 1
  spline S85 degree 3 poles (13.4093, 2.8655) (13.4093, 3.4396) (14.7588, 3.5216) (14.8408, 2.9475) knots 0 0 0 0 1 1 1 1
  spline S86 degree 3 poles (14.8408, 2.9475) (14.8557, 2.8208) (14.9228, 2.776) (15.1018, 2.7611) knots 0 0 0 0 1 1 1 1
  spline S87 degree 3 poles (15.1018, 2.7611) (15.3404, 2.7387) (15.3404, 2.7387) (15.2733, 2.9773) knots 0 0 0 0 1 1 1 1
  spline S88 degree 3 poles (15.2733, 2.9773) (15.1838, 3.283) (14.9974, 3.4843) (14.6992, 3.6111) knots 0 0 0 0 1 1 1 1
  spline S89 degree 3 poles (14.6992, 3.6111) (14.4307, 3.7229) (13.8343, 3.7453) (13.5882, 3.6409) knots 0 0 0 0 1 1 1 1
  spline S90 degree 3 poles (5.0213, 3.5514) (4.9467, 3.3427) (3.955, 0.7629) (3.9029, 0.6361) knots 0 0 0 0 1 1 1 1
  spline S91 degree 3 poles (3.9029, 0.6361) (3.8507, 0.5168) (3.8805, 0.5019) (4.0967, 0.5243) knots 0 0 0 0 1 1 1 1
  spline S92 degree 3 poles (4.0967, 0.5243) (4.3278, 0.5467) (4.3502, 0.5765) (4.4919, 1.0164) knots 0 0 0 0 1 1 1 1
  line L26 (4.4919, 1.0164) -> (4.641, 1.4861)
  line L27 (4.641, 1.4861) -> (5.2748, 1.4638)
  line L28 (5.2748, 1.4638) -> (5.9085, 1.4414)
  line L29 (5.9085, 1.4414) -> (6.0576, 0.9791)
  spline S93 degree 3 poles (6.0576, 0.9791) (6.1993, 0.5243) (6.2142, 0.5094) (6.4603, 0.5094) knots 0 0 0 0 1 1 1 1
  spline S94 degree 3 poles (6.4603, 0.5094) (6.6765, 0.5094) (6.7063, 0.5318) (6.6616, 0.6436) knots 0 0 0 0 1 1 1 1
  spline S95 degree 3 poles (6.6616, 0.6436) (6.6243, 0.7107) (6.3633, 1.419) (6.0726, 2.2019) knots 0 0 0 0 1 1 1 1
  line L30 (6.0726, 2.2019) -> (5.5432, 3.6409)
  line L31 (5.5432, 3.6409) -> (5.2971, 3.6409)
  spline S96 degree 3 poles (5.2971, 3.6409) (5.1629, 3.6409) (5.0362, 3.5962) (5.0213, 3.5514) knots 0 0 0 0 1 1 1 1
  spline S97 degree 3 poles (5.4984, 2.612) (5.5954, 2.2988) (5.6923, 1.9857) (5.7072, 1.926) knots 0 0 0 0 1 1 1 1
  spline S98 degree 3 poles (5.7072, 1.926) (5.7296, 1.8366) (5.6476, 1.8142) (5.2449, 1.8067) knots 0 0 0 0 1 1 1 1
  spline S99 degree 3 poles (5.2449, 1.8067) (4.8274, 1.8067) (4.7603, 1.8216) (4.805, 1.9186) knots 0 0 0 0 1 1 1 1
  spline S100 degree 3 poles (4.805, 1.9186) (4.8349, 1.9857) (4.9467, 2.2988) (5.0511, 2.612) knots 0 0 0 0 1 1 1 1
  spline S101 degree 3 poles (5.0511, 2.612) (5.1555, 2.9326) (5.2598, 3.1936) (5.2822, 3.1936) knots 0 0 0 0 1 1 1 1
  spline S102 degree 3 poles (5.2822, 3.1936) (5.3046, 3.1936) (5.4015, 2.9326) (5.4984, 2.612) knots 0 0 0 0 1 1 1 1
  line L32 (10.2479, 2.0975) -> (10.2554, 0.5467)
  line L33 (10.2554, 0.5467) -> (11.4036, 0.5467)
  line L34 (11.4036, 0.5467) -> (12.5518, 0.5467)
  line L35 (12.5518, 0.5467) -> (12.5518, 0.7331)
  line L36 (12.5518, 0.7331) -> (12.5518, 0.9195)
  line L37 (12.5518, 0.9195) -> (11.6049, 0.8896)
  line L38 (11.6049, 0.8896) -> (10.6505, 0.8673)
  line L39 (10.6505, 0.8673) -> (10.6505, 1.4414)
  line L40 (10.6505, 1.4414) -> (10.6505, 2.023)
  line L41 (10.6505, 2.023) -> (11.508, 1.9857)
  line L42 (11.508, 1.9857) -> (12.3654, 1.9559)
  line L43 (12.3654, 1.9559) -> (12.3654, 2.1423)
  line L44 (12.3654, 2.1423) -> (12.3654, 2.3361)
  line L45 (12.3654, 2.3361) -> (11.508, 2.3063)
  line L46 (11.508, 2.3063) -> (10.6505, 2.2839)
  line L47 (10.6505, 2.2839) -> (10.6505, 2.776)
  line L48 (10.6505, 2.776) -> (10.6505, 3.2681)
  line L49 (10.6505, 3.2681) -> (11.5825, 3.2681)
  line L50 (11.5825, 3.2681) -> (12.5145, 3.2681)
  line L51 (12.5145, 3.2681) -> (12.5145, 3.4545)
  line L52 (12.5145, 3.4545) -> (12.5145, 3.6409)
  line L53 (12.5145, 3.6409) -> (11.3812, 3.6409)
  line L54 (11.3812, 3.6409) -> (10.2405, 3.6409)
  line L55 (10.2405, 3.6409) -> (10.2479, 2.0975)
  constraint midpoint L1 L4.start
  constraint midpoint L0 L4.end
  constraint midpoint L2 L5.start
  constraint midpoint L3 L5.end
sketch "Sketch9" plane through (-1, 0, 0) normal (-1, 0, 0) x (0, -1, 0)
  line L0 (-6.1, 0) -> (1, 0)
  line L1 (1, 0) -> (1, 7.7)
  line L2 (1, 7.7) -> (-6.1, 7.7)
  line L3 (-6.1, 7.7) -> (-6.1, 0)
  line L4 (-5.0281, 2.0657) -> (0.041, 2.1577) construction
  line L5 (0.041, 2.1577) -> (-0.0305, 6.0943) construction
  line L6 (-0.0305, 6.0943) -> (-5.0995, 6.0023) construction
  line L7 (-5.0995, 6.0023) -> (-5.0281, 2.0657) construction
  line L8 (-2.55, 7.7) -> (-2.5022, 0) construction
  line L9 (-6.1, 3.85) -> (1, 3.85) construction
  dimension "d106" = 3
  text T0 "JR" font "Arial" height 3 align left top in box 5.0698 x 3.9372 at (-5.0281, 2.0657) x (0.999835, 0.018148) y (-0.018148, 0.999835) spacing 1
  constraint midpoint L2 L8.start
  constraint coincident L0 L8.end
  constraint midpoint L3 L9.start
  constraint midpoint L1 L9.end
sketch "Sketch10" plane through (21.04, 0, 0) normal (1, 0, 0) x (0, 1, 0)
  line L0 (-1, 0) -> (6.1, 0)
  line L1 (6.1, 0) -> (6.1, 7.7)
  line L2 (-0.1954, 2.5582) -> (5.2063, 2.5683) construction
  line L3 (5.2063, 2.5683) -> (5.2005, 5.6572) construction
  line L4 (5.2005, 5.6572) -> (-0.2011, 5.6471) construction
  line L5 (-0.2011, 5.6471) -> (-0.1954, 2.5582) construction
  line L6 (-0.4863, 3.9101) -> (6.1, 3.85) construction
  line L7 (2.5, 8) -> (2.5, 0) construction
  line L8 (6.1, 7.7) -> (-1, 7.7)
  line L9 (-1, 7.7) -> (-1, 0)
  dimension "d107" = 3
  text T0 "SA" font "Arial" height 3 align left top in box 5.4017 x 3.089 at (-0.1954, 2.5582) x (0.999998, 0.001871) y (-0.001871, 0.999998) spacing 1
  constraint midpoint L1 L6.end
  constraint coincident L0 L7.end
  constraint perpendicular L0 L7
extrude "Extrude12" add sketch "Sketch10" along normal blind 0.3 text T0
extrude "Extrude14" add sketch "Sketch9" along normal blind 0.3 text T0
sketch "Sketch12" plane through (0, 0, 8.2) normal (0, 0, 1) x (-1, 0, 0)
  line L0 (1, 0.4685) -> (0.5045, 1)
  line L1 (1, 1) -> (0.5045, 1)
  line L2 (1, 0.4685) -> (1, 1)
  line L3 (-5.33, -4.85) -> (-6.93, -4.85)
  line L4 (-6.93, -4.85) -> (-6.93, -0.25)
  line L5 (-6.93, -0.25) -> (-5.33, -0.25)
  line L6 (-5.33, -0.25) -> (-5.33, -4.85)
  line L7 (-7.18, -5.1) -> (-5.08, -5.1)
  line L8 (-5.08, -5.1) -> (-5.08, 0)
  line L9 (-5.08, 0) -> (-7.18, 0)
  line L10 (-7.18, 0) -> (-7.18, -5.1)
  line L11 (-19.63, -0.25) -> (-18.03, -0.25)
  line L12 (-18.03, -0.25) -> (-18.03, -4.85)
  line L13 (-18.03, -4.85) -> (-19.63, -4.85)
  line L14 (-19.63, -4.85) -> (-19.63, -0.25)
  line L15 (-17.78, 0) -> (-19.88, 0)
  line L16 (-19.88, 0) -> (-19.88, -5.1)
  line L17 (-19.88, -5.1) -> (-17.78, -5.1)
  line L18 (-17.78, -5.1) -> (-17.78, 0)
  line L19 (-10.41, -0.25) -> (-10.41, -4.85)
  line L20 (-10.41, -4.85) -> (-12.01, -4.85)
  line L21 (-12.01, -4.85) -> (-12.01, -0.25)
  line L22 (-12.01, -0.25) -> (-10.41, -0.25)
  line L23 (-10.16, -5.1) -> (-10.16, 0)
  line L24 (-10.16, 0) -> (-12.26, 0)
  line L25 (-12.26, 0) -> (-12.26, -5.1)
  line L26 (-12.26, -5.1) -> (-10.16, -5.1)
  line L27 (-15.49, -4.85) -> (-17.09, -4.85)
  line L28 (-17.09, -4.85) -> (-17.09, -0.25)
  line L29 (-17.09, -0.25) -> (-15.49, -0.25)
  line L30 (-15.49, -0.25) -> (-15.49, -4.85)
  line L31 (-15.24, -5.1) -> (-15.24, 0)
  line L32 (-15.24, 0) -> (-17.34, 0)
  line L33 (-17.34, 0) -> (-17.34, -5.1)
  line L34 (-17.34, -5.1) -> (-15.24, -5.1)
  line L35 (-1.85, -0.25) -> (-0.25, -0.25)
  line L36 (-0.25, -0.25) -> (-0.25, -4.85)
  line L37 (-0.25, -4.85) -> (-1.85, -4.85)
  line L38 (-1.85, -4.85) -> (-1.85, -0.25)
  line L39 (-2.1, -5.1) -> (0, -5.1)
  line L40 (0, -5.1) -> (0, 0)
  line L41 (0, 0) -> (-2.1, 0)
  line L42 (-2.1, 0) -> (-2.1, -5.1)
  line L43 (-14.55, -0.25) -> (-12.95, -0.25)
  line L44 (-12.95, -0.25) -> (-12.95, -4.85)
  line L45 (-12.95, -4.85) -> (-14.55, -4.85)
  line L46 (-14.55, -4.85) -> (-14.55, -0.25)
  line L47 (-14.8, 0) -> (-14.8, -5.1)
  line L48 (-14.8, -5.1) -> (-12.7, -5.1)
  line L49 (-12.7, -5.1) -> (-12.7, 0)
  line L50 (-12.7, 0) -> (-14.8, 0)
  line L51 (-7.87, -4.85) -> (-9.47, -4.85)
  line L52 (-9.47, -4.85) -> (-9.47, -0.25)
  line L53 (-9.47, -0.25) -> (-7.87, -0.25)
  line L54 (-7.87, -0.25) -> (-7.87, -4.85)
  line L55 (-7.62, 0) -> (-9.72, 0)
  line L56 (-9.72, 0) -> (-9.72, -5.1)
  line L57 (-9.72, -5.1) -> (-7.62, -5.1)
  line L58 (-7.62, -5.1) -> (-7.62, 0)
  line L59 (-2.79, -4.85) -> (-4.39, -4.85)
  line L60 (-4.39, -4.85) -> (-4.39, -0.25)
  line L61 (-4.39, -0.25) -> (-2.79, -0.25)
  line L62 (-2.79, -0.25) -> (-2.79, -4.85)
  line L63 (-4.64, -5.1) -> (-2.54, -5.1)
  line L64 (-2.54, -5.1) -> (-2.54, 0)
  line L65 (-2.54, 0) -> (-4.64, 0)
  line L66 (-4.64, 0) -> (-4.64, -5.1)
extrude "Extrude17" cut sketch "Sketch12" against normal blind 8 contours L0 L1 L2
extrude "Extrude19" add 1 faces at (20.6533, 3.4, 7.7) along direction (0, 0, 1) blind 0.3
extrude "Extrude20" cut 12 faces at (17.2567, 1.7833, 8.2) (19.7967, 1.7833, 8.2) (7.0967, 3.3167, 8.2) (0.0833, 3.3167, 8.2) (14.7167, 1.7833, 8.2) (10.2433, 3.3167, 8.2) (7.7033, 3.3167, 8.2) (4.5567, 3.3167, 8.2) (7.7033, 3.3167, 8.2) (7.0967, 3.3167, 8.2) (4.5567, 3.3167, 8.2) (0.0833, 3.3167, 8.2) along direction (0, 0, -1) blind 0.2
fillet "Fillet6" radius 0.2 1 faces at (20.57, 1.7833, 8)
sketch "Sketch13" plane through (0, 0, 0) normal (0, 0, 1) x (1, 0, 0)
extrude "Extrude22" add sketch "Sketch8" along normal blind 0.3 contours S0 S1 S2 S3 S4 S5 S6 S7 S8 S9 S10 S11 S12 S13 S14 S15 S16 S17 S18 | S19 S20 S21 S22 L6 L7 S23 S24 L8 L9 S25 S26 L10 L11 S27 S28 S29 S30 S31 S32 | S33 S34 S35 S36 S37 S38 S39 S40 S41 S42 S43 S44 S45 S46 S47 | L12 L13 L14 L15 L16 L17 S48 S49 L18 L19 S50 S51 S52 L20 L21 S53 S54 L22 L23 | S59 S60 S61 S62 S63 S64 S65 S66 S67 S68 S69 S70 S71 S72 | S73 S74 S75 S76 S77 S78 S79 S80 S81 S82 S83 S84 S85 S86 S87 S88 S89 | S90 S91 S92 L26 L27 L28 L29 S93 S94 S95 L30 L31 S96 | L32 L33 L34 L35 L36 L37 L38 L39 L40 L41 L42 L43 L44 L45 L46 L47 L48 L49 L50 L51 L52 L53 L54 L55